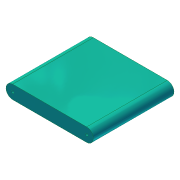
# Autodesk Inventor part: LateralConveyorRepresentation
Saved by Autodesk Inventor 2012 (Build 160160000, 160)
## iProperties
Created: 2013-01-22
Part Number: LateralConveyorRepresentation
Material: Default
Document SubType Name: Modeling
Designer: JesseK
Density: 1 g/cm^3
Mass: 4083.77 g
Surface Area: 2298.29 cm^2
Volume: 4083.77 cm^3
Author: JesseK
Autodesk Inventor part; units mm, degrees
ref_plane "YZ Plane" through (0, 0, 0) normal (1, 0, 0) x (0, 1, 0)
ref_plane "XZ Plane" through (0, 0, 0) normal (0, 1, 0) x (-1, 0, 0)
ref_plane "XY Plane" through (0, 0, 0) normal (0, 0, 1) x (1, 0, 0)
sketch "Sketch1" plane through (0, 0, 0) normal (0, 0, 1) x (1, 0, 0)
  arc A0 (0, 25.4) -> (0, -25.4) centre (0, 0) ccw
  arc A1 (279.4, -25.4) -> (279.4, 25.4) centre (279.4, 0) ccw
  line L0 (0, 25.4) -> (279.4, 25.4)
  line L1 (279.4, -25.4) -> (0, -25.4)
  dimension "d0" = 25.4
  dimension "d1" = 279.4
  constraints: 4 end point, 4 point on circle, 2 centre point, 2 horizontal, 2 tangent, 1 coincident, 1 equal radius
  measures "d0" radius of A0
  measures "d1" distance of A1.centre point (0, 0)
extrude "Extrusion1" add sketch "Sketch1" along normal blind 254
sketch "Sketch2" plane through (0, 0, 254) normal (0, 0, 1) x (1, 0, 0)
  arc A0 (0, 25.4) -> (0, -25.4) centre (0, 0) ccw projected
  arc A1 (279.4, -25.4) -> (279.4, 25.4) centre (279.4, 0) ccw projected
  circle A2 centre (0, 0) radius 4.7625
  circle A3 centre (279.4, 0) radius 4.7625
  dimension "d4" = 9.525
  constraints: 2 centre point, 2 coincident, 1 equal radius
  measures "d4" diameter of A2
extrude "Extrusion2" cut sketch "Sketch2" against normal through all
body "Solid1"
